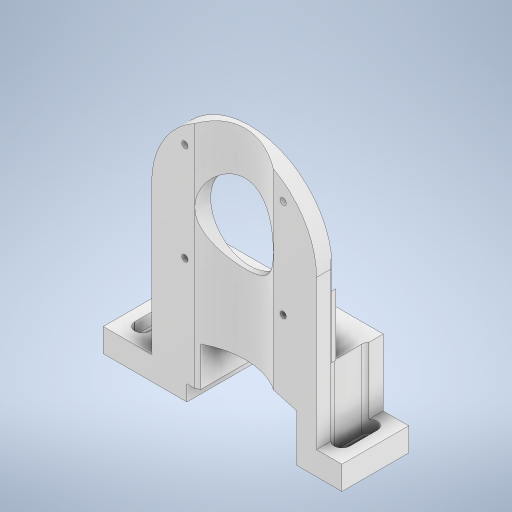
# Autodesk Inventor part: Rotator Mount - Klinger Motor
Saved by Autodesk Inventor 2024 (Build 280153000, 153)
## iProperties
Created: 2024-11-12
Part Number: Rotator Mount - Klinger Motor
Material: ABS Plastic
Document SubType Name: Modeling
Designer: Kemper Room 121
Density: 1.06 g/cm^3
Appearance: Smooth - White
Mass: 329.624 g
Surface Area: 519.697 cm^2
Volume: 310.966 cm^3
Author: Kemper Room 121
Autodesk Inventor part; units mm, degrees
ref_plane "YZ Plane" through (0, 0, 0) normal (1, 0, 0) x (0, 1, 0)
ref_plane "XZ Plane" through (0, 0, 0) normal (0, 1, 0) x (-1, 0, 0)
ref_plane "XY Plane" through (0, 0, 0) normal (0, 0, 1) x (1, 0, 0)
sketch "Sketch1" plane through (0, 0, 0) normal (0, 0, 1) x (1, 0, 0)
  circle A0 centre (0, 0) radius 50
  line L0 (0, 0) -> (0, -50)
  line L1 (0, -50) -> (0, -110)
  line L2 (0, -110) -> (5.4, -110)
  line L3 (0, -110) -> (-20, -110)
  line L4 (5.4, -110) -> (56.2, -110)
  line L5 (-20, -110) -> (-70.8, -110)
  line L6 (56.2, -110) -> (68.7, -110)
  line L7 (-70.8, -110) -> (-83.3, -110)
  line L8 (-83.3, -110) -> (-83.3, -102.5)
  line L9 (-83.3, -102.5) -> (-83.3, -95)
  line L10 (-83.3, -95) -> (-52.5, -95)
  circle A1 centre (0, 0) radius 52.5
  line L11 (-52.5, 0) -> (-52.5, -95)
  line L12 (52.5, 0) -> (52.5, -95)
  line L13 (52.5, -95) -> (68.7, -95)
  line L14 (68.7, -95) -> (68.7, -110)
  circle A2 centre (0, 0) radius 25
  dimension "d0" = 100
  dimension "d1" = 5.4
  dimension "d2" = 20
  dimension "d3" = 60
  dimension "d4" = 50.8
  dimension "d5" = 50.8
  dimension "d6" = 12.5
  dimension "d7" = 12.5
  dimension "d8" = 7.5
  dimension "d9" = 7.5
  dimension "d10" = 105
  dimension "d11" = 0
  dimension "d23" = 50
  constraints: 30 end point, 6 horizontal, 4 perpendicular, 3 coincident, 3 vertical, 2 centre point, 2 point on circle, 2 point on line, 1 tangent, 1 vertical alignment, 2 other
  measures "d1" distance of L1.end L2.end
  measures "d2" distance of L1.end L3.end
  measures "d3" distance of L0.end L1.end
  measures "d4" distance of L2.end L4.end
  measures "d5" distance of L3.end L5.end
  measures "d6" distance of L4.end L6.end
  measures "d7" distance of L5.end L7.end
  measures "d8" distance of L7.end L8.end
  measures "d9" distance of L8.end L9.end
  measures "d10" diameter of A1
  measures "d11" distance of L11.end L10.end
  measures "d23" diameter of A2
extrude "Extrusion1" add sketch "Sketch1" along normal blind 10 contours A0 | A1 L12 L13 L14 L6 L4 L2 L1 | L1 L3 L5 L7 L8 L9 L10 L11 A1 | A1
sketch "Sketch2" plane through (0, 0, 0) normal (0, 0, -1) x (-1, 0, 0)
  line L0 (52.5, -95) -> (83.3, -95) projected
  line L1 (52.5, 0) -> (52.5, -95) projected
  arc A0 (52.5, 0) -> (-52.5, 0) centre (0, 0) ccw projected
  line L2 (-52.5, -95) -> (-52.5, 0) projected
  line L3 (-68.7, -95) -> (-52.5, -95) projected
  line L4 (-68.7, -110) -> (-68.7, -95) projected
  line L5 (83.3, -110) -> (-68.7, -110) projected
  line L6 (83.3, -95) -> (83.3, -110) projected
  line L7 (-22.5, -110) -> (22.5, -110)
  line L8 (22.5, -110) -> (22.5, -75)
  line L9 (22.5, -75) -> (-22.5, -75)
  line L10 (-22.5, -75) -> (-22.5, -110)
  line L11 (-52.5, -52.5) -> (52.5, -52.5)
  line L12 (52.5, -52.5) -> (52.5, 52.5)
  line L13 (52.5, 52.5) -> (-52.5, 52.5)
  line L14 (-52.5, 52.5) -> (-52.5, -52.5)
  line L15 (83.3, -110) -> (-68.7, -110) projected
  line L16 (-22.5, -110) -> (-68.7, -110)
  line L17 (-68.7, -110) -> (-68.7, -95)
  line L18 (-68.7, -95) -> (-52.5, -95) projected
  line L19 (-68.7, -95) -> (-52.5, -95)
  line L20 (-52.5, -95) -> (-52.5, -52.5)
  line L21 (52.5, -52.5) -> (52.5, -95)
  line L22 (52.5, -95) -> (83.3, -95)
  line L23 (83.3, -95) -> (83.3, -110)
  line L24 (83.3, -110) -> (22.5, -110)
  point P0 (0, -110)
  point P1 (0, 52.5)
  point P2 (52.5, 0)
  dimension "d14" = 35
  dimension "d15" = 0
  dimension "d16" = 45
  dimension "d17" = 105
  dimension "d18" = 105
  dimension "d19" = 0
  dimension "d20" = 0
  constraints: 32 end point, 5 perpendicular, 4 horizontal, 4 parallel, 3 midpoint, 1 collinear, 1 point on line
  measures "d14" distance of L7.end L8.end
  measures "d15" horizontal distance of point (0, 0) point (0, -110)
  measures "d16" distance of L8.end L9.end
  measures "d17" distance of L11.end L12.end
  measures "d18" distance of L12.end L13.end
  measures "d19" horizontal distance of point (0, 0) point (0, 52.5)
  measures "d20" vertical distance of point (52.5, 0) point (0, 0)
extrude "Extrusion2" add sketch "Sketch2" along normal blind 32.5 contours L0 L6 L5 L8 L9 L10 L4 L3 L2 L11 L1
sketch "Sketch3" plane through (0, 0, -32.5) normal (0, 0, -1) x (-1, 0, 0)
  line L0 (22.5, -75) -> (22.5, -110) projected
  line L1 (22.5, -110) -> (83.3, -110) projected
  line L2 (83.3, -110) -> (83.3, -95) projected
  line L3 (83.3, -95) -> (52.5, -95) projected
  line L4 (52.5, -95) -> (52.5, -52.5) projected
  line L5 (52.5, -52.5) -> (-52.5, -52.5) projected
  line L6 (-52.5, -52.5) -> (-52.5, -95) projected
  line L7 (-52.5, -95) -> (-68.7, -95) projected
  line L8 (-68.7, -95) -> (-68.7, -110) projected
  line L9 (-68.7, -110) -> (-22.5, -110) projected
  line L10 (-22.5, -110) -> (-22.5, -75) projected
  line L11 (-22.5, -75) -> (22.5, -75) projected
  line L12 (-68.7, -110) -> (78.3, -110)
  line L13 (78.3, -110) -> (78.3, -52.5)
  line L14 (78.3, -52.5) -> (-68.7, -52.5)
  line L15 (-68.7, -52.5) -> (-68.7, -110)
  line L16 (22.5, -75) -> (-22.5, -75) projected
  line L17 (-22.5, -110) -> (22.5, -110)
  line L18 (22.5, -110) -> (22.5, -75)
  line L19 (22.5, -75) -> (-22.5, -75)
  line L20 (-22.5, -75) -> (-22.5, -110)
  line L21 (52.5, -95) -> (78.3, -95)
  line L22 (78.3, -95) -> (78.3, -52.5)
  line L23 (78.3, -52.5) -> (52.5, -52.5)
  line L24 (52.5, -52.5) -> (52.5, -95)
  line L25 (-52.5, -95) -> (-68.7, -95)
  line L26 (-68.7, -95) -> (-68.7, -52.5)
  line L27 (-68.7, -52.5) -> (-52.5, -52.5)
  line L28 (-52.5, -52.5) -> (-52.5, -95)
  point P0 (0, 0)
  constraints: 32 end point, 8 parallel, 4 horizontal, 4 perpendicular
extrude "Extrusion3" cut sketch "Sketch3" against normal through all contours L0 L12 L10 L11
sketch "Sketch4" plane through (-83.3, -95, 10) normal (0, 1, 0) x (1, 0, 0)
  line L0 (0, 42.5) -> (0, 0) projected
  line L1 (30.8, 0) -> (0, 0) projected
  line L2 (30.8, 0) -> (30.8, 42.5) projected
  line L3 (0, 42.5) -> (30.8, 42.5) projected
  line L4 (135.8, 42.5) -> (135.8, 0) projected
  line L5 (152, 0) -> (135.8, 0) projected
  line L6 (152, 42.5) -> (152, 0) projected
  line L7 (135.8, 42.5) -> (152, 42.5) projected
  arc A0 (9.325, 12.5) -> (15.675, 12.5) centre (12.5, 12.5) ccw
  arc A1 (142.675, 30) -> (136.325, 30) centre (139.5, 30) ccw
  arc A2 (15.675, 30) -> (9.325, 30) centre (12.5, 30) ccw
  arc A3 (136.325, 12.5) -> (142.675, 12.5) centre (139.5, 12.5) ccw
  line L8 (15.675, 30) -> (15.675, 12.5)
  line L9 (9.325, 12.5) -> (9.325, 30)
  line L10 (142.675, 30) -> (142.675, 12.5)
  line L11 (136.325, 12.5) -> (136.325, 30)
  point P0 (83.3, 10)
  point P1 (0, 21.25)
  point P2 (152, 21.25)
  point P3 (143.9, 0)
  dimension "d28" = 6.35
  dimension "d29" = 6.35
  dimension "d30" = 12.5
  dimension "d31" = 12.5
  dimension "d72" = 6.35
  dimension "d73" = 0
  dimension "d74" = 6.35
  dimension "d75" = 12.5
  dimension "d76" = 12.5
  dimension "d77" = 12.5
  dimension "d78" = 12.5
  constraints: 8 end point, 8 point on circle, 4 centre point, 3 midpoint, 2 parallel
  measures "d28" diameter of A0
  measures "d29" diameter of A1
  measures "d30" distance from line of L0 A0.centre
  measures "d31" distance from line of L6 A1.centre
  measures "d72" diameter of A2
  measures "d73" horizontal distance of A3.centre A1.centre
  measures "d74" diameter of A3
  measures "d75" distance from line of L1 A0.centre
  measures "d76" distance from line of L3 A2.centre
  measures "d77" distance from line of L7 A1.centre
  measures "d78" vertical distance of point (143.9, 0) A3.centre
extrude "Extrusion4" cut sketch "Sketch4" against normal through all contours L9 A2 L8 A0 | L10 A3 L11 A1
sketch "Sketch5" plane through (-83.3, -95, 10) normal (0, 1, 0) x (1, 0, 0)
  arc A0 (9.325, 12.5) -> (15.675, 12.5) centre (12.5, 12.5) ccw projected
  line L0 (0, 42.5) -> (0, 0) projected
  line L1 (30.8, 0) -> (0, 0) projected
  line L2 (30.8, 0) -> (30.8, 42.5) projected
  line L3 (0, 42.5) -> (30.8, 42.5) projected
  arc A1 (142.675, 30) -> (136.325, 30) centre (139.5, 30) ccw projected
  line L4 (135.8, 42.5) -> (135.8, 0) projected
  line L5 (152, 0) -> (135.8, 0) projected
  line L6 (152, 42.5) -> (152, 0) projected
  line L7 (135.8, 42.5) -> (152, 42.5) projected
  arc A2 (7.5, 12.5) -> (17.5, 12.5) centre (12.5, 12.5) ccw
  circle A3 centre (139.5, 30) radius 5
  arc A4 (136.325, 12.5) -> (142.675, 12.5) centre (139.5, 12.5) ccw projected
  line L8 (136.325, 12.5) -> (136.325, 30) projected
  line L9 (142.675, 30) -> (142.675, 12.5) projected
  arc A5 (15.675, 30) -> (9.325, 30) centre (12.5, 30) ccw projected
  line L10 (15.675, 30) -> (15.675, 12.5) projected
  line L11 (9.325, 12.5) -> (9.325, 30) projected
  arc A6 (17.5, 29.2188) -> (7.4393, 30) centre (12.5, 30) ccw
  arc A7 (135.8, 15.863) -> (144.5, 12.5) centre (139.5, 12.5) ccw
  line L12 (17.5, 30) -> (17.5, 12.5)
  line L13 (7.4393, 12.5) -> (7.4393, 30)
  line L14 (144.5, 30) -> (134.5, 30)
  line L15 (134.5, 30) -> (134.5, 12.5)
  line L16 (144.5, 12.5) -> (144.5, 30)
  line L17 (15.675, 30) -> (17.5, 30)
  line L18 (7.5, 12.5) -> (7.4393, 12.5)
  line L19 (134.5, 12.5) -> (135.8, 12.5)
  point P0 (83.3, 10)
  point P1 (135.8, 26.637)
  point P2 (135.8, 9.137)
  dimension "d35" = 10
  dimension "d34" = 10
  constraints: 20 end point, 7 point on circle, 4 coincident, 4 parallel, 3 centre point, 3 point on line, 2 horizontal, 2 perpendicular, 3 other
  measures "d34" diameter of A2
extrude "Extrusion5" cut sketch "Sketch5" against normal blind 7.5 contours L11 A5 L10 A0 | L14 A1 | L14 A3 L9 | A1 L14 L4 A3 | L9 A3 L8 L14 | L8 A3 L4 L14 | L9 A4 L8 A3 | A3 L16 A7 L4 L8 A4 L9 | L14 A3 L4 | L4 A3 L14 | L4 A7 L15 A3 | A7 L19 L4 | L4 L19 A7 | L18 L13 A6 L12 A2
sketch "Sketch6" plane through (52.5, -95, 10) normal (0, 1, 0) x (1, 0, 0)
  arc A0 (8.7, 30) -> (0, 33.363) centre (3.7, 30) ccw projected
  line L0 (0, 9.137) -> (0, 0) projected
  line L1 (16.2, 0) -> (0, 0) projected
  line L2 (16.2, 42.5) -> (16.2, 0) projected
  line L3 (0, 42.5) -> (16.2, 42.5) projected
  circle A1 centre (3.7, 30) radius 5
  line L4 (0, 42.5) -> (0, 33.363) projected
  line L5 (8.7, 30) -> (8.7, 12.5) projected
  arc A2 (0, 9.137) -> (8.7, 12.5) centre (3.7, 12.5) ccw projected
  circle A3 centre (3.7, 12.5) radius 5
  arc A4 (0, 9.137) -> (8.7, 12.5) centre (3.7, 12.5) ccw projected
  line L6 (8.7, 12.5) -> (-1.3, 12.5)
  line L7 (-1.3, 12.5) -> (-1.3, 30)
  line L8 (-1.3, 30) -> (8.7, 30)
  line L9 (8.7, 30) -> (8.7, 12.5)
  point P0 (-52.5, 10)
  point P1 (0, 33.363)
  point P2 (8.7, 30)
  constraints: 8 end point, 2 coincident, 2 parallel, 1 centre point, 1 concentric, 1 horizontal, 1 perpendicular, 4 other
extrude "Extrusion6" cut sketch "Sketch6" along normal through all contours L8 A1 A0 | L5 A3 L7 A1 | A1 L8 | L6 A3 | A2 A3 L6
sketch "Sketch7" plane through (0, 0, 10) normal (0, 0, 1) x (1, 0, 0)
  line L0 (22.5, -75) -> (22.5, -110) projected
  line L1 (22.5, -110) -> (68.7, -110) projected
  line L2 (68.7, -110) -> (68.7, -95) projected
  line L3 (68.7, -95) -> (52.5, -95) projected
  line L4 (52.5, -95) -> (52.5, 0) projected
  arc A0 (52.5, 0) -> (-52.5, 0) centre (0, 0) ccw projected
  line L5 (-52.5, 0) -> (-52.5, -95) projected
  line L6 (-52.5, -95) -> (-83.3, -95) projected
  line L7 (-83.3, -95) -> (-83.3, -110) projected
  line L8 (-83.3, -110) -> (-22.5, -110) projected
  line L9 (-22.5, -110) -> (-22.5, -75) projected
  line L10 (-22.5, -75) -> (22.5, -75) projected
  circle A1 centre (0, 0) radius 25 projected
  line L11 (40, -110) -> (40, -80)
  line L12 (40, -80) -> (22.5, -75)
  line L13 (22.5, -75) -> (-22.5, -75) projected
  line L14 (22.5, -75) -> (22.5, -110)
  line L15 (68.7, -110) -> (22.5, -110) projected
  line L16 (40, -110) -> (22.5, -110)
  line L17 (0, -110) -> (-30, -110)
  line L18 (-30, -110) -> (-30, -100)
  line L19 (-30, -100) -> (-17.5, -100)
  line L20 (-17.5, -100) -> (-17.5, -75)
  line L21 (-17.5, -75) -> (22.5, -75)
  line L22 (0, -110) -> (22.5, -110)
  point P0 (-22.5, -100)
  dimension "d40" = 40
  dimension "d41" = 30
  dimension "d44" = 30
  dimension "d45" = 10
  dimension "d46" = 12.5
  constraints: 20 end point, 4 perpendicular, 4 point on line, 1 collinear, 1 horizontal, 1 parallel, 1 vertical
  measures "d40" distance from line of L11 point (0, 0)
  measures "d41" distance of L11.start L11.end
  measures "d44" distance of L17.start L17.end
  measures "d45" distance of L17.end L18.end
  measures "d46" distance of L18.end L19.end
extrude "Extrusion7" cut sketch "Sketch7" against normal through all contours L12 L11 L1 L0 | L8 L18 L19 L9
sketch "Sketch8" plane through (0, 0, 0) normal (0, 0, -1) x (-1, 0, 0)
  circle A0 centre (0, 0) radius 25 projected
  line L0 (-51.8699, -52.5) -> (52.5, -52.5) projected
  line L1 (52.5, 0) -> (52.5, -52.5) projected
  arc A1 (52.5, 0) -> (-51.8699, 8.1096) centre (0, 0) ccw projected
  circle A2 centre (0, 0) radius 52.5
  circle A3 centre (0, 0) radius 50
  circle A4 centre (0, 0) radius 53.5
  circle A5 centre (0, 0) radius 55.5
  line L2 (52.5, -10.2956) -> (52.5, -18)
  line L3 (52.5, 0) -> (52.5, -95) projected
  line L4 (-52.5, -10.2956) -> (-52.5, -18)
  line L5 (-52.5, -95) -> (-52.5, 0) projected
  line L6 (-51.8699, 8.1096) -> (-51.8699, -52.5) projected
  point P0 (-52.5, -52.5)
  point P1 (18, -52.5)
  point P2 (52.5, -18)
  point P3 (10.2956, -52.5)
  point P4 (-18, -52.5)
  point P5 (-10.2956, -52.5)
  point P6 (-51.8699, -19.7425)
  point P7 (-51.8699, -13.106)
  dimension "d47" = 100
  dimension "d48" = 52.5
  dimension "d49" = 107
  dimension "d50" = 111
  constraints: 4 centre point, 4 coincident, 4 end point, 4 point on circle, 3 point on line, 1 concentric
  measures "d47" diameter of A3
  measures "d48" radius of A1
  measures "d49" diameter of A4
  measures "d50" diameter of A5
extrude "Extrusion8" add sketch "Sketch8" along normal blind 3 contours L6 A5 L0 | A5 L6 A4 L0 | A5 L1 L0 | L0 A4 L1 A5
sketch "Sketch9" plane through (0, 0, 10) normal (0, 0, 1) x (1, 0, 0)
  line L0 (40, -110) -> (68.7, -110) projected
  line L1 (68.7, -110) -> (68.7, -95) projected
  line L2 (68.7, -95) -> (52.5, -95) projected
  line L3 (52.5, -95) -> (52.5, 0) projected
  arc A0 (52.5, 0) -> (-52.5, 0) centre (0, 0) ccw projected
  line L4 (-52.5, 0) -> (-52.5, -95) projected
  line L5 (-52.5, -95) -> (-83.3, -95) projected
  line L6 (-83.3, -95) -> (-83.3, -110) projected
  line L7 (-83.3, -110) -> (-30, -110) projected
  line L8 (-22.5, -100) -> (-22.5, -75) projected
  line L9 (-22.5, -75) -> (22.5, -75) projected
  circle A1 centre (0, 0) radius 25 projected
  circle A2 centre (0, 0) radius 44.25
  circle A3 centre (31.2895, 31.2895) radius 2
  line L10 (0, 0) -> (43.4168, 43.4168)
  line L11 (0, 0) -> (62.8571, 0)
  circle A4 centre (-31.2895, 31.2895) radius 2
  circle A5 centre (-31.2895, -31.2895) radius 2
  circle A6 centre (31.2895, -31.2895) radius 2
  line L12 (40, -80) -> (40, -110) projected
  line L13 (-30, -110) -> (-30, -100) projected
  line L14 (-30, -100) -> (-22.5, -100) projected
  line L15 (22.5, -75) -> (40, -80) projected
  dimension "d53" = 88.5
  dimension "d55" = 45
  dimension "d56" = 4
  dimension "d59" = 360
  constraints: 4 centre point, 4 end point, 1 coincident, 1 horizontal, 1 point on line, 12 other
  measures "d55" angle of L11 L10
  measures "d56" diameter of A3
extrude "Extrusion9" cut sketch "Sketch9" against normal through all contours L10 A2 A3 | A3 A2 L10 | A3 L10 A2 | A6 A2 | A2 A6 | A2 L10 A3 | A4 A2 | A2 A4 | A5 A2 | A2 A5
sketch "Sketch10" plane through (-83.3, -110, -32.5) normal (0, -1, 0) x (1, 0, 0)
  line L0 (135.1699, 32.5) -> (30.8, 32.5) projected
  line L1 (30.8, 32.5) -> (30.8, 42.5) projected
  line L2 (135.8, 42.5) -> (30.8, 42.5) projected
  line L3 (135.8, 33.363) -> (135.8, 42.5) projected
  line L4 (105.8, 35.5) -> (60.8, 35.5)
  line L5 (105.8, 0) -> (105.8, 42.5) projected
  line L6 (60.8, 42.5) -> (60.8, 0) projected
  arc A0 (105.8, 42.5) -> (83.3, 35.5) centre (83.3, 75.1607) ccw
  line L7 (108.3, 35.5) -> (58.3, 35.5)
  line L8 (58.3, 35.5) -> (58.3, 42.5)
  line L9 (108.3, 35.5) -> (108.3, 42.5)
  arc A1 (83.3, 35.5) -> (58.3, 42.5) centre (83.3, 83.6429) ccw
  circle A2 centre (83.3, 83.6429) radius 48.1429
  point P0 (83.3, 32.5)
  point P1 (83.3, 42.5)
  point P2 (58.3, 42.5)
  point P3 (83.3, 35.5)
  dimension "d63" = 45
  dimension "d64" = 0
  dimension "d65" = 3
  dimension "d66" = 50
  dimension "d68" = 0
  dimension "d71" = 0
  constraints: 8 end point, 6 point on circle, 3 centre point, 3 midpoint, 2 horizontal, 2 perpendicular, 2 point on line, 1 coincident, 1 concentric, 1 other
  measures "d63" distance of L4.start L4.end
  measures "d64" horizontal distance of point (83.3, 42.5) A0.end
  measures "d65" distance between parallel lines of L0 L4
  measures "d66" distance of L7.start L7.end
  measures "d68" distance between parallel lines of L4 L7
  measures "d71" horizontal distance of point (83.3, 42.5) A1.start
extrude "Extrusion10" cut sketch "Sketch10" against normal through all contours A2 L6 A0 | A0 L2 L5 A1 | L5 L2 A1 | A2 L2 L6
equation "\"d0\" = Motor_Attachment_Mount_OD"
equation "\"d10\" = Motor_W"
equation "\"d23\" = Motor_Thru_Hole_D"
equation "\"d17\" = Motor_W"
equation "\"d18\" = Motor_L"
equation "\"d29\" = d28"
equation "\"d72\" = d28"
equation "\"d74\" = d29"
equation "\"d75\" = d30"
equation "\"d76\" = d30"
equation "\"d77\" = d31"
equation "\"d78\" = d31"
equation "\"d47\" = Motor_Attachment_Mount_OD"
equation "\"d53\" = Motor_Attachment_Mount_D"
equation "\"d56\" = Motor_Attachment_Hole_D"
equation "\"Motor_L\" = 105"
equation "\"Motor_W\" = 105"
equation "\"Motor_Attachment_Mount_D\" = 88.5"
equation "\"Motor_Attachment_Hole_D\" = 4"
equation "\"Motor_Attachment_Mount_OD\" = 100"
equation "\"Motor_Thru_Hole_D\" = 50"
equation "\"Cable_Plate_Thickness\" = 5"
equation "\"Cable_Connector_D1\" = 26.825"
equation "\"Cable_Connector_D2\" = 18.75"
equation "\"Encoder_L\" = 103"
equation "\"Motor_Thickness\" = 28"
equation "\"Encoder_Thickness\" = 28"
equation "\"Cable_Plate_L\" = 103.25"
equation "\"Cable_Plate_W\" = 28"
equation "\"Motor_Drive_L\" = 22"
equation "\"Post_Tighten_D\" = 4"
equation "\"Motor_Mount_Wall_Thickness\" = 5"
equation "\"Motor_Alignment_D\" = 22"
equation "\"Motor_Mount_Countersink_D\" = 6"
equation "\"Post_D\" = 12.7"
equation "\"Cage_Mount_Rotator_Thickness\" = 7.9"
equation "\"Motor_Mount_Hole_Spacing\" = 31"
equation "\"Motor_Drive_D\" = 5"
equation "\"Post_Tighten_Countersink_Depth\" = 4.5"
equation "\"Cage_Mount_Thickness\" = 12.7"
equation "\"Motor_Mount_Countersink\" = 3"
equation "\"Post_Tighten_Countersink_D\" = 7.5"
equation "\"Tabletop_Hole_Spacing\" = 25.4"
equation "\"Structure_Wall\" = 4"
equation "\"Motor_Mount_Hole_D\" = 3"
equation "\"Tabletop_Hole_D\" = 6.35"
equation "\"Thick_Wall\" = 6"
equation "\"Drive_Output_Offset\" = 29"
equation "\"Cage_Mount_W\" = 71.1"
equation "\"Cage_Mount_L\" = 71.1"
equation "\"Moderate_Wall\" = 4.5"
equation "\"Cage_Mount_Hole_D\" = 6"
equation "\"Thin_Wall\" = 3"
body "Solid1"
